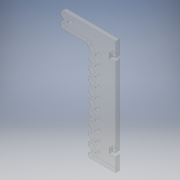
# Autodesk Inventor part: primary_holder
Saved by Autodesk Inventor 2016 (Build 200138000, 138)
## iProperties
Created: 2018-04-27
Part Number: primary_holder
Material: Polycarbonate, Clear
Document SubType Name: Modeling
Designer: Phil Erle
Density: 1.2 g/cm^3
Appearance: Polycarbonate - Clear
Author: Phil Erle
Autodesk Inventor part; units mm, degrees
ref_plane "YZ Plane" through (0, 0, 0) normal (1, 0, 0) x (0, 1, 0)
ref_plane "XZ Plane" through (0, 0, 0) normal (0, 1, 0) x (-1, 0, 0)
ref_plane "XY Plane" through (0, 0, 0) normal (0, 0, 1) x (1, 0, 0)
sketch "Sketch1" plane through (0, 0, 0) normal (0, 1, 0) x (-1, 0, 0)
  line L0 (0, 0) -> (70, 0)
  line L1 (70, 0) -> (70, -20)
  line L2 (70, -20) -> (35, -20)
  line L3 (35, -20) -> (35, -145)
  line L4 (35, -145) -> (0, -145)
  line L5 (0, -145) -> (0, 0)
  dimension "d0" = 35
  dimension "d1" = 145
  dimension "d2" = 70
  dimension "d3" = 20
  constraints: 12 end point, 4 perpendicular, 1 horizontal, 1 vertical
  measures "d0" distance of L3.end L4.end
  measures "d1" distance between parallel lines of L4 L0
  measures "d2" distance of L0.start L0.end
  measures "d3" distance of L0.end L1.end
extrude "Extrusion1" add sketch "Sketch1" along normal blind 5
sketch "Sketch2" plane through (0, 5, 0) normal (0, 1, 0) x (1, 0, 0)
  line L0 (-70, 20) -> (-70, 0) projected
  circle A0 centre (-70, 10) radius 4
  line L1 (-35, 145) -> (-35, 20) projected
  circle A1 centre (-35, 64.5) radius 4
  circle A2 centre (-35, 76.5) radius 4
  circle A3 centre (-35, 88.5) radius 4
  circle A4 centre (-35, 100.5) radius 4
  circle A5 centre (-35, 112.5) radius 4
  circle A6 centre (-35, 124.5) radius 4
  circle A7 centre (-35, 136.5) radius 4
  circle A8 centre (-35, 52.5) radius 4
  circle A9 centre (-35, 40.5) radius 4
  circle A10 centre (-35, 28.5) radius 4
  line L2 (0, 17.75) -> (0, 22.25)
  line L3 (0, 22.25) -> (-5, 22.25)
  line L4 (-5, 22.25) -> (-5, 23.5)
  line L5 (-5, 23.5) -> (-8.2, 23.5)
  line L6 (-8.2, 23.5) -> (-8.2, 16.5)
  line L7 (-8.2, 16.5) -> (-5, 16.5)
  line L8 (0, 17.75) -> (-5, 17.75)
  line L9 (-5, 17.75) -> (-5, 16.5)
  line L10 (0, 0) -> (0, 145) projected
  line L11 (0, 127.25) -> (-5, 127.25)
  line L12 (-5, 127.25) -> (-5, 128.5)
  line L13 (-5, 128.5) -> (-8.2, 128.5)
  line L14 (-8.2, 128.5) -> (-8.2, 121.5)
  line L15 (-8.2, 121.5) -> (-5, 121.5)
  line L16 (-5, 121.5) -> (-5, 122.75)
  line L17 (-5, 122.75) -> (0, 122.75)
  line L18 (0, 122.75) -> (0, 127.25)
  line L19 (-25, 28.5) -> (-25, 136.5) construction
  circle A11 centre (-25, 28.5) radius 1.5
  circle A12 centre (-25, 40.5) radius 1.5
  circle A13 centre (-25, 52.5) radius 1.5
  circle A14 centre (-25, 64.5) radius 1.5
  circle A15 centre (-25, 76.5) radius 1.5
  circle A16 centre (-25, 88.5) radius 1.5
  circle A17 centre (-25, 100.5) radius 1.5
  circle A18 centre (-25, 112.5) radius 1.5
  circle A19 centre (-25, 124.5) radius 1.5
  circle A20 centre (-25, 136.5) radius 1.5
  circle A21 centre (-60, 10) radius 1.5
  point P0 (-8.2, 125)
  point P1 (0, 125)
  point P2 (-8.2, 20)
  point P3 (0, 20)
  dimension "d6" = 8
  dimension "d7" = 8
  dimension "d8" = 8
  dimension "d9" = 8
  dimension "d11" = 8
  dimension "d12" = 8
  dimension "d13" = 8
  dimension "d14" = 8
  dimension "d15" = 8.5
  dimension "d16" = 12
  dimension "d17" = 12
  dimension "d18" = 12
  dimension "d19" = 12
  dimension "d20" = 12
  dimension "d21" = 12
  dimension "d22" = 8
  dimension "d23" = 8
  dimension "d24" = 12
  dimension "d25" = 12
  dimension "d26" = 12
  dimension "d27" = 8
  dimension "d28" = 7
  dimension "d29" = 3.2
  dimension "d30" = 4.5
  dimension "d31" = 5
  dimension "d32" = 3.2
  dimension "d33" = 5
  dimension "d34" = 7
  dimension "d35" = 4.5
  dimension "d36" = 20
  dimension "d37" = 20
  dimension "d38" = 3
  dimension "d39" = 3
  dimension "d40" = 3
  dimension "d41" = 3
  dimension "d42" = 3
  dimension "d43" = 3
  dimension "d44" = 3
  dimension "d45" = 3
  dimension "d46" = 3
  dimension "d47" = 3
  dimension "d48" = 10
  dimension "d52" = 3
  dimension "d53" = 10
  constraints: 32 end point, 22 centre point, 13 horizontal alignment, 10 perpendicular, 6 midpoint, 5 point on line, 3 horizontal, 2 coincident, 2 vertical, 1 vertical alignment, 22 other
  measures "d6" diameter of A0
  measures "d7" diameter of A1
  measures "d8" diameter of A2
  measures "d9" diameter of A3
  measures "d11" diameter of A4
  measures "d12" diameter of A5
  measures "d13" diameter of A6
  measures "d14" diameter of A7
  measures "d15" distance of point (-35, 145) A7.centre
  measures "d16" distance of A7.centre A6.centre
  measures "d17" distance of A6.centre A5.centre
  measures "d18" distance of A5.centre A4.centre
  measures "d19" distance of A4.centre A3.centre
  measures "d20" distance of A3.centre A2.centre
  measures "d21" distance of A2.centre A1.centre
  measures "d22" diameter of A8
  measures "d23" diameter of A9
  measures "d24" distance of A1.centre A8.centre
  measures "d25" distance of A8.centre A9.centre
  measures "d26" distance of A9.centre A10.centre
  measures "d27" diameter of A10
  measures "d28" distance of L13.end L14.end
  measures "d29" distance of L12.end L13.end
  measures "d30" distance between parallel lines of L11 L17
  measures "d31" distance of L11.start L11.end
  measures "d32" distance of L6.end L7.end
  measures "d33" distance of L2.start L8.end
  measures "d34" distance of L5.end L6.end
  measures "d35" distance between parallel lines of L8 L3
  measures "d36" distance of L10.end point (0, 125)
  measures "d37" distance of L10.start point (0, 20)
  measures "d38" diameter of A11
  measures "d39" diameter of A12
  measures "d40" diameter of A13
  measures "d41" diameter of A14
  measures "d42" diameter of A15
  measures "d43" diameter of A16
  measures "d44" diameter of A17
  measures "d45" diameter of A18
  measures "d46" diameter of A19
  measures "d47" diameter of A20
  measures "d52" diameter of A21
  measures "d53" distance of A0.centre A21.centre
extrude "Extrusion2" cut sketch "Sketch2" against normal blind 5
fillet "Fillet1" radius 3 4 edges at (-35, 2.5, -145) (-35, 2.5, -20) (-70, 2.5, -20) (-70, 2.5, 0)
body "Solid1"
